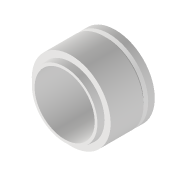
# Autodesk Inventor part: 00_microscope_turret
Saved by Autodesk Inventor 2022 (Build 260153000, 153)
## iProperties
Created: 2023-01-08
Part Number: 00_microscope_turret
Material: Generisch
Document SubType Name: Modeling
Designer: diederichbenedict
Density: 1 g/cm^3
Appearance: Vorgabe
Author: diederichbenedict
Autodesk Inventor part; units mm, degrees
ref_plane "YZ Plane" through (0, 0, 0) normal (1, 0, 0) x (0, 1, 0)
ref_plane "XZ Plane" through (0, 0, 0) normal (0, 1, 0) x (-1, 0, 0)
ref_plane "XY Plane" through (0, 0, 0) normal (0, 0, 1) x (1, 0, 0)
sketch "Skizze1" plane through (0, 0, 0) normal (1, 0, 0) x (0, 1, 0)
  line L0 (23.95, 0) -> (23.95, 4)
  line L1 (23.95, 4) -> (22.5358, 5.4142)
  line L2 (22.5358, 5.4142) -> (23.95, 6.8284)
  line L3 (23.95, 6.8284) -> (23.95, 26.8284)
  line L4 (23.95, 26.8284) -> (20.25, 26.8284)
  line L5 (20.25, 26.8284) -> (20.25, 30.8284)
  line L6 (20.25, 30.8284) -> (18.25, 30.8284)
  line L7 (18.25, 30.8284) -> (18.25, 0)
  line L8 (18.25, 0) -> (23.95, 0)
  line L9 (0, -6.1657) -> (0, 36.9941) projected
  point P0 (0, 0)
  dimension "d0" = 4
  dimension "d1" = 2
  dimension "d2" = 135
  dimension "d3" = 20
  dimension "d4" = 23.95
  dimension "d5" = 20.25
  dimension "d6" = 4
  dimension "d7" = 2
  constraints: 18 end point, 6 perpendicular, 2 point on line, 1 vertical
  measures "d0" distance of L0.start L0.end
  measures "d1" distance of L0.end L1.end
  measures "d2" angle of L1 L0
  measures "d3" distance of L2.end L3.end
  measures "d4" distance of L0.start point (0, 0)
  measures "d5" distance from line of point (0, 0) L5
  measures "d6" distance from line of L4 L6.end
  measures "d7" distance between parallel lines of L5 L7
revolve "Umdrehung1" add sketch "Skizze1" angle 360 about axis through (0, 0, -10) along (0, 0, 1)
sketch "Skizze2" plane through (0, 0, 26.8284) normal (0, 0, 1) x (1, 0, 0)
  circle A0 centre (0, 0) radius 20.25 projected
  circle A1 centre (0, 0) radius 23.95 projected
extrude "Extrusion1" cut sketch "Skizze2" along normal up to surface (4 mm away) draft 5
